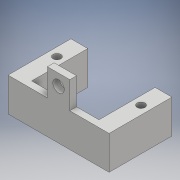
# Autodesk Inventor part: Raket_Arme_Motor
Saved by Autodesk Inventor 2018 (Build 220112000, 112)
## iProperties
Created: 2017-08-14
Part Number: Raket_Arme_Motor
Material: Generic
Document SubType Name: Modeling
Designer: andre
Density: 1 g/cm^3
Appearance: Default
Author: andre
## iProperties of the stored document Raket_Arme_Motor_3DPrint.ipt
Created: 2017-08-14
Part Number: Raket_Arme_Motor_3DPrint
Material: Generic
Document SubType Name: Modeling
Designer: andre
Density: 1 g/cm^3
Appearance: Default
Author: andre
Autodesk Inventor part; units mm, degrees
ref_plane "YZ Plane" through (0, 0, 0) normal (1, 0, 0) x (0, 1, 0)
ref_plane "XZ Plane" through (0, 0, 0) normal (0, 1, 0) x (-1, 0, 0)
ref_plane "XY Plane" through (0, 0, 0) normal (0, 0, 1) x (1, 0, 0)
sketch "Sketch1" plane through (0, 0, 0) normal (0, 1, 0) x (-1, 0, 0)
  line L0 (0, 0) -> (10, 0)
  line L1 (10, 0) -> (10, -27)
  line L2 (10, -27) -> (0, -27)
  line L3 (0, -27) -> (0, 0)
  dimension "d0" = 10
  dimension "d1" = 27
  constraints: 8 end point, 2 parallel, 1 horizontal, 1 perpendicular
  measures "d0" distance of L1.end L2.end
  measures "d1" distance of L0.end L1.end
extrude "Extrusion1" add sketch "Sketch1" along normal blind 10
sketch "Sketch2" plane through (0, 10, 0) normal (0, 1, 0) x (1, 0, 0)
  line L0 (-10, 27) -> (-10, 0) projected
  line L1 (-10, 0) -> (-10, 5)
  circle A0 centre (-5, 5) radius 2.55
  point P0 (0, 0)
  dimension "d4" = 5
  dimension "d5" = 5.1
  constraints: 2 end point, 1 centre point, 1 point on line
  measures "d4" distance of L0.end L1.end
  measures "d5" diameter of A0
extrude "Extrusion2" cut sketch "Sketch2" against normal blind 10
sketch "Sketch4" plane through (0, 10, 0) normal (0, 1, 0) x (1, 0, 0)
  line L0 (0, 27) -> (-10, 27) projected
  line L1 (-10, 27) -> (-10, 0) projected
  line L2 (0, 27) -> (-10, 27)
  line L3 (-10, 27) -> (-10, 0)
  line L4 (-10, 0) -> (0, 0)
  line L5 (0, 0) -> (0, 27)
  point P0 (0, 0)
  dimension "d13" = 27
  constraints: 8 end point, 2 parallel, 1 horizontal, 1 perpendicular, 1 point on line
  measures "d13" distance of L3.end L2.end
extrude "Extrusion4" cut sketch "Sketch4" against normal blind 7
sketch "Sketch5" plane through (0, 3, 0) normal (0, 1, 0) x (1, 0, 0)
  line L0 (-10, 27) -> (0, 27) projected
  line L1 (-5, 27) -> (17.5, 27)
  line L2 (17.5, 27) -> (17.5, 12)
  line L3 (17.5, 12) -> (-5, 12)
  line L4 (-5, 12) -> (-5, 27)
  line L5 (-5, 27) -> (-27.5, 27)
  line L6 (-27.5, 27) -> (-27.5, 12)
  line L7 (-27.5, 12) -> (-5, 12)
  line L8 (-5, 12) -> (-5, 27)
  point P0 (0, 0)
  dimension "d16" = 22.5
  dimension "d17" = 15
  dimension "d18" = 22.5
  constraints: 16 end point, 4 parallel, 2 horizontal, 2 perpendicular, 1 midpoint
  measures "d16" distance of L2.end L3.end
  measures "d17" distance of L1.end L2.end
  measures "d18" distance of L7.end L6.end
extrude "Extrusion5" add sketch "Sketch5" against normal blind 3
sketch "Sketch6" plane through (0, 3, 0) normal (0, 1, 0) x (1, 0, 0)
  line L0 (17.5, 12) -> (-27.5, 12) projected
  line L1 (-5, 12) -> (10, 12)
  line L2 (10, 12) -> (10, 27)
  line L3 (-27.5, 27) -> (17.5, 27) projected
  line L4 (-5, 12) -> (-20, 12)
  line L5 (-27.5, 12) -> (-10, 12) projected
  line L6 (-20, 12) -> (-20, 27)
  line L7 (-20, 12) -> (-27.5, 12)
  line L8 (-27.5, 12) -> (-27.5, 27)
  line L9 (-27.5, 27) -> (-20, 27)
  line L10 (-20, 27) -> (-20, 12)
  line L11 (10, 12) -> (17.5, 12)
  line L12 (17.5, 12) -> (17.5, 27)
  line L13 (17.5, 27) -> (10, 27)
  line L14 (10, 27) -> (10, 12)
  point P0 (0, 0)
  dimension "d21" = 15
  dimension "d22" = 15
  constraints: 24 end point, 4 parallel, 4 perpendicular, 3 point on line, 2 horizontal, 1 midpoint
  measures "d21" distance of L1.start L1.end
  measures "d22" distance of L1.start L4.end
extrude "Extrusion6" add sketch "Sketch6" along normal blind 25 contours L0 L2 L3 L12 | L6 L0 L8 L3
sketch "Sketch7" plane through (17.5, 0, -27) normal (0, 0, -1) x (-1, 0, 0)
  line L0 (37.5, 3) -> (7.5, 3) projected
  line L1 (7.5, 3) -> (0, 3)
  line L2 (0, 0) -> (0, 28) projected
  line L3 (3.75, 3) -> (3.75, 18)
  line L4 (37.5, 3) -> (44.9906, 3)
  line L5 (41.2453, 3) -> (41.2453, 18)
  circle A0 centre (3.75, 18) radius 1.75
  circle A1 centre (41.2453, 18) radius 1.75
  point P0 (17.5, 0)
  dimension "d25" = 15
  dimension "d26" = 15
  dimension "d27" = 3.5
  dimension "d28" = 3.5
  constraints: 8 end point, 2 centre point, 2 coincident, 2 horizontal, 2 midpoint, 2 vertical, 1 point on line
  measures "d25" distance of L3.start L3.end
  measures "d26" distance of L5.start L5.end
  measures "d27" diameter of A0
  measures "d28" diameter of A1
extrude "Extrusion7" cut sketch "Sketch7" against normal blind 25
body "Solid1"
